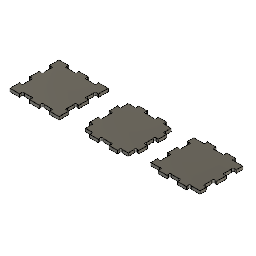
a5_box (Autodesk Fusion 360 design; units mm, degrees)
Autodesk Fusion 360 part; units mm, degrees
note: some values were not read from the file. Set by a fixed rule: which sketch regions a step uses.
sketch "Sketch1" plane through (0, 0, 0) normal (0, 0, 1) x (1, 0, 0)
  line L0 (-100.34, 0) -> (0, 0)
  line L1 (0, 0) -> (0, 70.41)
  line L2 (0, 70.41) -> (-100.34, 70.41)
  line L3 (-100.34, 70.41) -> (-100.34, 0)
  dimension "d1" = 100.34
  dimension "d2" = 70.41
  constraint horizontal L0
  constraint vertical L1
  constraint horizontal L2
  constraint vertical L3
  constraint coincident L0.end L1.start
  measures "d1" distance of L0.start L0.end
  measures "d2" distance of L0.start L2.end
  measures "d104" distance of L0.end
extrude "Extrude1" add sketch "Sketch1" along normal blind 1.58 makes body 1
sketch "Sketch3" plane through (0, 0, 0) normal (0, 0, 1) x (1, 0, 0)
  line L0 (10, 25) -> (35, 25)
  line L1 (35, 25) -> (35, 0)
  line L2 (35, 0) -> (10, 0)
  line L3 (10, 0) -> (10, 25)
  line L4 (10, 25) -> (11.58, 25)
  line L5 (11.58, 25) -> (11.58, 0)
  line L6 (11.58, 0) -> (10, 0)
  line L7 (10, 0) -> (10, 25)
  line L8 (10, 25) -> (35, 25)
  line L9 (35, 25) -> (35, 23.42)
  line L10 (35, 23.42) -> (10, 23.42)
  line L11 (10, 23.42) -> (10, 25)
  line L12 (35, 25) -> (33.42, 25)
  line L13 (33.42, 25) -> (33.42, 0)
  line L14 (33.42, 0) -> (35, 0)
  line L15 (35, 0) -> (35, 25)
  line L16 (10, 0) -> (35, 0)
  line L17 (35, 0) -> (35, 1.58)
  line L18 (35, 1.58) -> (10, 1.58)
  line L19 (10, 1.58) -> (10, 0)
  dimension "d5" = 25
  dimension "d6" = 25
  dimension "d14" = 1.58
  dimension "d15" = 1.58
  dimension "d16" = 1.58
  dimension "d17" = 1.58
  constraint horizontal L0
  constraint vertical L1
  constraint horizontal L2
  constraint vertical L3
  constraint horizontal L4
  constraint vertical L5
  constraint horizontal L6
  constraint vertical L7
  constraint horizontal L8
  constraint vertical L9
  constraint horizontal L10
  constraint vertical L11
  constraint horizontal L12
  constraint vertical L13
  constraint horizontal L14
  constraint vertical L15
  constraint horizontal L16
  constraint vertical L17
  constraint horizontal L18
  constraint vertical L19
  measures "d5" distance of L0.start L0.end
  measures "d6" distance of L0.start L2.end
  measures "d14" distance of L0.start L4.end
  measures "d15" distance of L0.start L10.end
  measures "d16" distance of L0.end L12.end
  measures "d17" distance of L2.end L18.end
extrude "Extrude3" add sketch "Sketch3" along normal blind 25 separate body contours L0 L3 L4 L5 L7 L8 L10 L11 | L0 L5 L8 L10 L13 | L3 L5 L7 L10 L18 | L0 L1 L8 L9 L10 L12 L13 L15 | L2 L3 L5 L6 L7 L16 L18 L19 | L1 L10 L13 L15 L18 | L2 L5 L13 L16 L18 | L1 L2 L13 L14 L15 L16 L17 L18 makes body 2
extrude "Extrude4" add sketch "Sketch3" along normal blind 1.58 contours L5 L10 L13 L18 bodies 2
sketch "Sketch5" plane through (0, 0, 25) normal (0, 0, 1) x (-1, 0, 0)
  line L0 (-11.58, -1.58) -> (-11.58, -23.42)
  line L1 (-11.58, -23.42) -> (-33.42, -23.42)
  line L2 (-33.42, -23.42) -> (-33.42, -1.58)
  line L3 (-33.42, -1.58) -> (-11.58, -1.58)
  line L4 (-10, -25) -> (-10, 0)
  line L5 (-10, 0) -> (-35, 0)
  line L6 (-35, 0) -> (-35, -25)
  line L7 (-35, -25) -> (-10, -25)
  line L8 (-10, -25) -> (-35, -25)
  line L9 (-35, -25) -> (-35, 0)
  line L10 (-35, 0) -> (-10, 0)
  line L11 (-10, 0) -> (-10, -25)
  constraint horizontal L8
  constraint vertical L9
  constraint horizontal L10
  constraint vertical L11
  constraint coincident L5.end L6.start
  constraint coincident L4.start L7.end
extrude "Extrude5" add sketch "Sketch5" against normal blind 1.58 contours L0 L1 L2 L3 bodies 2
sketch "Sketch6" plane through (0, 0, 25) normal (0, 0, 1) x (-1, 0, 0)
  line L0 (-10, -25) -> (-10, 0)
  line L1 (-10, 0) -> (-35, 0)
  line L2 (-35, 0) -> (-35, -25)
  line L3 (-35, -25) -> (-10, -25)
  line L4 (-14.9996, 0) -> (-14.9996, -1.58)
  line L5 (-19.9996, -1.58) -> (-19.9996, 0)
  line L6 (-25.0019, 0) -> (-25.0019, -1.58)
  line L7 (-30.0019, -1.58) -> (-30.0019, 0)
  line L8 (-14.9996, -1.58) -> (-19.9996, -1.58)
  line L9 (-25.0019, -1.58) -> (-30.0019, -1.58)
  line L10 (-11.58, -1.58) -> (-33.42, -1.58)
  line L11 (-14.7996, 0) -> (-14.7996, -1.78)
  line L12 (-14.7996, -1.78) -> (-20.1996, -1.78)
  line L13 (-20.1996, -1.78) -> (-20.1996, 0)
  line L14 (-24.8, 0) -> (-24.8, -1.78)
  line L15 (-24.8, -1.78) -> (-30.2, -1.78)
  line L16 (-30.2, -1.78) -> (-30.2, 0)
  line L17 (-55.1361, -25) -> (-80.1361, -25)
  line L18 (-80.1361, -25) -> (-80.1361, 0)
  line L19 (-80.1361, 0) -> (-55.1361, 0)
  line L20 (-55.1361, 0) -> (-55.1361, -25)
  line L21 (-60.1361, 0) -> (-65.1361, 0)
  line L22 (-65.1361, 0) -> (-65.1361, -1.58)
  line L23 (-65.1361, -1.58) -> (-60.1361, -1.58)
  line L24 (-60.1361, -1.58) -> (-60.1361, 0)
  line L25 (-70.1361, 0) -> (-75.1361, 0)
  line L26 (-75.1361, 0) -> (-75.1361, -1.58)
  line L27 (-75.1361, -1.58) -> (-70.1361, -1.58)
  line L28 (-70.1361, -1.58) -> (-70.1361, 0)
  line L29 (-67.6361, -25) -> (-67.6361, 0) construction
  line L30 (-55.1361, -12.5) -> (-80.1361, -12.5) construction
  line L31 (-70.1361, -23.42) -> (-70.1361, -25)
  line L32 (-75.1361, -23.42) -> (-70.1361, -23.42)
  line L33 (-75.1361, -25) -> (-75.1361, -23.42)
  line L34 (-65.1361, -25) -> (-65.1361, -23.42)
  line L35 (-65.1361, -23.42) -> (-60.1361, -23.42)
  line L36 (-60.1361, -23.42) -> (-60.1361, -25)
  line L37 (-55.1361, -25) -> (-80.1361, 0) construction
  line L38 (-80.1361, -25) -> (-55.1361, 0) construction
  line L39 (-55.1361, -5) -> (-56.7161, -5)
  line L40 (-55.1361, -15) -> (-56.7161, -15)
  line L41 (-56.7161, -20) -> (-55.1361, -20)
  line L42 (-56.7161, -15) -> (-56.7161, -20)
  line L43 (-56.7161, -10) -> (-55.1361, -10)
  line L44 (-56.7161, -5) -> (-56.7161, -10)
  line L45 (-80.1361, -10) -> (-78.5561, -10)
  line L46 (-78.5561, -5) -> (-80.1361, -5)
  line L47 (-78.5561, -10) -> (-78.5561, -5)
  line L48 (-80.1361, -20) -> (-78.5561, -20)
  line L49 (-78.5561, -20) -> (-78.5561, -15)
  line L50 (-78.5561, -15) -> (-80.1361, -15)
  point P0 (-55.1361, -12.5)
  point P1 (-80.1361, -12.5)
  dimension "d24" = 1.78
  dimension "d25" = 0.2
  dimension "d26" = 5
  dimension "d27" = 5.4
  dimension "d28" = 1.78
  dimension "d29" = 5
  dimension "d30" = 5.4
  dimension "d31" = 25
  dimension "d32" = 25
  dimension "d33" = 5
  dimension "d34" = 1.58
  dimension "d35" = 5
  dimension "d36" = 1.58
  dimension "d37" = 5
  dimension "d38" = 5
  constraint coincident L1 L4.start
  constraint coincident L1 L5.end
  constraint perpendicular L1 L5
  constraint coincident L1 L6.start
  constraint coincident L1 L7.end
  constraint perpendicular L1 L7
  constraint perpendicular L5 L8
  constraint perpendicular L7 L9
  constraint coincident L4.end L10
  constraint coincident L6.end L10
  constraint perpendicular L6 L9
  constraint perpendicular L4 L8
  constraint coincident L1 L11.start
  constraint perpendicular L10 L11
  constraint perpendicular L11 L12
  constraint coincident L1 L13.end
  constraint perpendicular L1 L13
  constraint coincident L1 L14.start
  constraint perpendicular L10 L14
  constraint perpendicular L14 L15
  constraint coincident L1 L16.end
  constraint perpendicular L1 L16
  constraint horizontal L17
  constraint vertical L18
  constraint horizontal L19
  constraint vertical L20
  constraint horizontal L21
  constraint vertical L22
  constraint horizontal L23
  constraint vertical L24
  constraint coincident L19 L21.start
  constraint horizontal L25
  constraint vertical L26
  constraint horizontal L27
  constraint vertical L28
  constraint coincident L19 L25.start
  constraint midpoint L17 L29.start
  constraint midpoint L19 L29.end
  constraint midpoint L20 P0
  constraint midpoint L18 P1
  constraint symmetric L21.start L30 L36.end
  constraint symmetric L21.end L30 L34.start
  constraint symmetric L22.end L30 L34.end
  constraint symmetric L23.end L30 L35.end
  constraint symmetric L25.start L30 L31.end
  constraint symmetric L25.end L30 L33.start
  constraint symmetric L26.end L30 L32.start
  constraint symmetric L27.end L30 L31.start
  constraint symmetric L29.start L37 P0
  constraint symmetric L31.start L37 L43.start
  constraint symmetric L31.end L37 L43.end
  constraint symmetric L32.start L37 L39.end
  constraint symmetric L33.start L37 L39.start
  constraint symmetric L34.start L37 L40.start
  constraint symmetric L34.end L37 L40.end
  constraint symmetric L35.end L37 L41.start
  constraint symmetric L36.end L37 L41.end
  constraint symmetric L29.start L38 P1
  constraint symmetric L31.start L38 L49.end
  constraint symmetric L31.end L38 L50.end
  constraint symmetric L32.start L38 L48.end
  constraint symmetric L33.start L38 L48.start
  constraint symmetric L34.start L38 L45.start
  constraint symmetric L34.end L38 L45.end
  constraint symmetric L35.end L38 L46.start
  constraint symmetric L36.end L38 L46.end
  measures "d24" distance of L11.start L11.end
  measures "d25" distance of L4 L11
  measures "d26" distance of L4.end L5.start
  measures "d27" distance of L11.end L12.end
  measures "d28" distance of L14.start L14.end
  measures "d29" distance of L6.end L7.start
  measures "d30" distance of L14.end L15.end
  measures "d31" distance of L17.start L17.end
  measures "d32" distance of L17.start L19.end
  measures "d33" distance of L21.start L21.end
  measures "d34" distance of L21.start L23.end
  measures "d35" distance of L20 L24
  measures "d36" distance of L25.start L27.end
  measures "d37" distance of L25.start L25.end
  measures "d38" distance of L22 L28
extrude "Extrude6" add sketch "Sketch6" along normal blind 1.58 separate body contours L17 L18 L19 L20 L22 L23 L24 L26 L27 L28 L31 L32 L33 L34 L35 L36 L39 L40 L41 L42 L43 L44 L45 L46 L47 L48 L49 L50 makes body 3
sketch "Sketch9" plane through (0, 0, 26.58) normal (0, 0, 1) x (-1, 0, 0)
  line L0 (-75.1361, -25) -> (-75.1361, -23.42)
  line L1 (-75.1361, -23.42) -> (-70.1361, -23.42)
  line L2 (-70.1361, -23.42) -> (-70.1361, -25)
  line L3 (-70.1361, -25) -> (-65.1361, -25)
  line L4 (-65.1361, -25) -> (-65.1361, -23.42)
  line L5 (-65.1361, -23.42) -> (-60.1361, -23.42)
  line L6 (-60.1361, -23.42) -> (-60.1361, -25)
  line L7 (-60.1361, -25) -> (-55.1361, -25)
  line L8 (-55.1361, -25) -> (-55.1361, -20)
  line L9 (-55.1361, -20) -> (-56.7161, -20)
  line L10 (-56.7161, -20) -> (-56.7161, -15)
  line L11 (-56.7161, -15) -> (-55.1361, -15)
  line L12 (-55.1361, -15) -> (-55.1361, -10)
  line L13 (-55.1361, -10) -> (-56.7161, -10)
  line L14 (-56.7161, -10) -> (-56.7161, -5)
  line L15 (-56.7161, -5) -> (-55.1361, -5)
  line L16 (-55.1361, -5) -> (-55.1361, 0)
  line L17 (-55.1361, 0) -> (-60.1361, 0)
  line L18 (-60.1361, 0) -> (-60.1361, -1.58)
  line L19 (-60.1361, -1.58) -> (-65.1361, -1.58)
  line L20 (-65.1361, -1.58) -> (-65.1361, 0)
  line L21 (-65.1361, 0) -> (-70.1361, 0)
  line L22 (-70.1361, 0) -> (-70.1361, -1.58)
  line L23 (-70.1361, -1.58) -> (-75.1361, -1.58)
  line L24 (-75.1361, -1.58) -> (-75.1361, 0)
  line L25 (-75.1361, 0) -> (-80.1361, 0)
  line L26 (-80.1361, 0) -> (-80.1361, -5)
  line L27 (-80.1361, -5) -> (-78.5561, -5)
  line L28 (-78.5561, -5) -> (-78.5561, -10)
  line L29 (-78.5561, -10) -> (-80.1361, -10)
  line L30 (-80.1361, -10) -> (-80.1361, -15)
  line L31 (-80.1361, -15) -> (-78.5561, -15)
  line L32 (-78.5561, -15) -> (-78.5561, -20)
  line L33 (-78.5561, -20) -> (-80.1361, -20)
  line L34 (-80.1361, -20) -> (-80.1361, -25)
  line L35 (-80.1361, -25) -> (-75.1361, -25)
  line L36 (-60.1361, -23.42) -> (-61.3154, -24.5992) construction
  line L37 (-60.1361, -23.42) -> (-58.4685, -23.42) construction
  circle A0 centre (-60.5571, -23.8409) radius 0.5953
  line L38 (-62.6361, -23.42) -> (-62.6361, -1.58) construction
  line L39 (-67.6361, -25) -> (-67.6361, 0) construction
  line L40 (-55.1361, -12.5) -> (-80.1361, -12.5) construction
  line L41 (-80.1361, 0) -> (-55.1361, -25) construction
  circle A1 centre (-64.7152, -23.8409) radius 0.5953
  circle A2 centre (-74.7152, -23.8409) radius 0.5953
  circle A3 centre (-70.5571, -23.8409) radius 0.5953
  circle A4 centre (-60.5571, -1.1591) radius 0.5953
  circle A5 centre (-64.7152, -1.1591) radius 0.5953
  circle A6 centre (-70.5571, -1.1591) radius 0.5953
  circle A7 centre (-74.7152, -1.1591) radius 0.5953
  circle A8 centre (-56.2952, -19.5791) radius 0.5953
  circle A9 centre (-56.2952, -15.4209) radius 0.5953
  circle A10 centre (-56.2952, -9.5791) radius 0.5953
  circle A11 centre (-56.2952, -5.4209) radius 0.5953
  circle A12 centre (-78.9771, -15.4209) radius 0.5953
  circle A13 centre (-78.9771, -19.5791) radius 0.5953
  circle A14 centre (-78.9771, -9.5791) radius 0.5953
  circle A15 centre (-78.9771, -5.4209) radius 0.5953
  dimension "d41" = 135
  dimension "d42" = 1.1906
  dimension "d43" = 0.5953
  constraint horizontal L37
  constraint coincident L5.end L6.start
  constraint coincident L36 A0.centre
  constraint midpoint L5 L38.start
  constraint midpoint L19 L38.end
  constraint midpoint L3 L39.start
  constraint midpoint L21 L39.end
  constraint midpoint L12 L40.start
  constraint midpoint L30 L40.end
  constraint coincident L25.end L26.start
  constraint coincident L7.end L8.start
  constraint symmetric A0 L38 A1
  constraint symmetric A0 L39 A2
  constraint symmetric L39 A1 A3
  constraint symmetric A0 L40 A4
  constraint symmetric L40 A1 A5
  constraint symmetric L40 A2 A7
  constraint symmetric L40 A3 A6
  constraint symmetric A0 L41 A8
  constraint symmetric L41 A1 A9
  constraint symmetric L41 A2 A11
  constraint symmetric L41 A3 A10
  constraint symmetric L39 A8 A13
  constraint symmetric L39 A9 A12
  constraint symmetric L39 A10 A14
  constraint symmetric L39 A11 A15
  measures "d41" angle of L36 L37
  measures "d42" diameter of A0
  measures "d43" distance of L5.end A0.centre
extrude "Extrude7" cut sketch "Sketch9" against normal up to surface (1.58 mm away) contours L0 A2 | L0 L1 A2 | L1 A2 | L32 L33 A13 | L33 A13 | L1 A3 | L1 L2 A3 | L32 A13 | L2 A3 | L31 L32 A12 | L32 A12 | L31 A12 | L4 A1 | L4 L5 A1 | L5 A1 | L28 L29 A14 | L29 A14 | L28 A14 | L5 A0 | L5 L6 A0 | L27 L28 A15 | L28 A15 | L6 A0 | L27 A15 | L9 A8 | L9 L10 A8 | L23 L24 A7 | L24 A7 | L10 A8 | L23 A7 | L10 A9 | L10 L11 A9 | L22 L23 A6 | L23 A6 | L11 A9 | L22 A6 | L19 L20 A5 | L20 A5 | L13 A10 | L13 L14 A10 | L19 A5 | L14 A10 | L18 L19 A4 | L19 A4 | L14 A11 | L14 L15 A11 | L18 A4 | L15 A11 bodies 3
sketch "Sketch10" plane through (0, 0, 0) normal (0, 0, 1) x (1, 0, 0)
  line L0 (115.2, 23.42) -> (115.2, 0)
  line L1 (115.2, 0) -> (90.2, 0)
  line L2 (90.2, 0) -> (90.2, 19.6)
  line L3 (90.2, 25) -> (95.6, 25)
  line L4 (95.6, 25) -> (95.6, 23.42)
  line L5 (95.6, 23.42) -> (90.2, 23.42)
  line L6 (90.2, 23.42) -> (90.2, 25)
  line L7 (100, 25) -> (105.4, 25)
  line L8 (105.4, 25) -> (105.4, 23.42)
  line L9 (105.4, 23.42) -> (100, 23.42)
  line L10 (100, 23.42) -> (100, 25)
  line L11 (109.8, 25) -> (115.2, 25)
  line L12 (115.2, 25) -> (115.2, 23.42)
  line L13 (115.2, 23.42) -> (109.8, 23.42)
  line L14 (109.8, 23.42) -> (109.8, 25)
  line L15 (90.2, 12.5) -> (115.2, 12.5) construction
  line L16 (102.7, 25) -> (102.7, 0) construction
  line L17 (91.78, 5.4) -> (91.78, 0)
  line L18 (90.2, 5.4) -> (91.78, 5.4)
  line L19 (91.78, 9.8) -> (90.2, 9.8)
  line L20 (91.78, 15.2) -> (91.78, 9.8)
  line L21 (90.2, 15.2) -> (91.78, 15.2)
  line L22 (91.78, 19.6) -> (90.2, 19.6)
  line L23 (91.78, 25) -> (91.78, 19.6)
  line L24 (109.8, 1.58) -> (115.2, 1.58)
  line L25 (109.8, 0) -> (109.8, 1.58)
  line L26 (105.4, 1.58) -> (105.4, 0)
  line L27 (100, 1.58) -> (105.4, 1.58)
  line L28 (100, 0) -> (100, 1.58)
  line L29 (95.6, 1.58) -> (95.6, 0)
  line L30 (90.2, 1.58) -> (95.6, 1.58)
  line L31 (113.62, 19.6) -> (113.62, 25)
  line L32 (115.2, 19.6) -> (113.62, 19.6)
  line L33 (113.62, 15.2) -> (115.2, 15.2)
  line L34 (113.62, 9.8) -> (113.62, 15.2)
  line L35 (115.2, 9.8) -> (113.62, 9.8)
  line L36 (113.62, 5.4) -> (115.2, 5.4)
  line L37 (113.62, 0) -> (113.62, 5.4)
  line L38 (90.2, 23.42) -> (90.2, 25)
  line L39 (90.2, 19.6) -> (90.2, 23.42)
  line L40 (115.2, 25) -> (115.2, 23.42)
  line L41 (109.8, 25) -> (115.2, 25)
  line L42 (105.4, 25) -> (109.8, 25)
  line L43 (90.2, 25) -> (95.6, 25)
  line L44 (100, 25) -> (105.4, 25)
  line L45 (95.6, 25) -> (100, 25)
  point P0 (102.7, 12.5)
  dimension "d46" = 25
  dimension "d47" = 25
  dimension "d48" = 5.4
  dimension "d49" = 1.58
  dimension "d50" = 5.4
  dimension "d51" = 1.58
  dimension "d52" = 5.4
  dimension "d53" = 1.58
  dimension "d57" = 360
  dimension "d73" = 4.4
  dimension "d74" = 4.4
  constraint horizontal L43
  constraint vertical L0
  constraint horizontal L1
  constraint vertical L2
  constraint horizontal L3
  constraint vertical L4
  constraint horizontal L5
  constraint vertical L6
  constraint horizontal L7
  constraint vertical L8
  constraint horizontal L9
  constraint vertical L10
  constraint coincident L7.start L43
  constraint horizontal L11
  constraint vertical L12
  constraint horizontal L13
  constraint vertical L14
  constraint coincident L11.start L43
  constraint midpoint L1 L16.end
  constraint midpoint L16 P0
  constraint collinear L0 L12
  constraint coincident L2 L15.start
  constraint coincident L0 L15.end
  constraint coincident L16.start L43
  measures "d46" distance of L3.start L11.end
  measures "d47" distance of L3.start L1.end
  measures "d48" distance of L3.start L3.end
  measures "d49" distance of L3.start L5.end
  measures "d50" distance of L7.start L7.end
  measures "d51" distance of L7.start L9.end
  measures "d52" distance of L11.start L11.end
  measures "d53" distance of L11.start L13.end
  measures "d73" distance of L4 L10
  measures "d74" distance of L8 L14
extrude "Extrude8" add sketch "Sketch10" along normal blind 1.58 separate body contours L0 L1 L2 L4 L5 L8 L9 L10 L13 L14 L17 L18 L19 L20 L21 L22 L23 L24 L25 L26 L27 L28 L29 L30 L31 L32 L33 L34 L35 L36 L37 L42 L45 makes body 4
sketch "Sketch12" plane through (0, 0, 0) normal (0, 0, 1) x (1, 0, 0)
  line L0 (100, 23.42) -> (100, 25) construction
  circle A0 centre (114.041, 20.0209) radius 0.5953
  circle A1 centre (91.3591, 20.0209) radius 0.5953
  line L1 (95.6, 23.42) -> (97.2763, 23.42) construction
  line L2 (102.7, 25.8483) -> (102.7, 0.1169) construction
  circle A2 centre (104.9791, 23.8409) radius 0.5953
  circle A3 centre (114.041, 4.9791) radius 0.5953
  circle A4 centre (110.221, 1.1591) radius 0.5953
  circle A5 centre (100.421, 1.1591) radius 0.5953
  circle A6 centre (91.3591, 4.9791) radius 0.5953
  circle A7 centre (91.3591, 10.2209) radius 0.5953
  circle A8 centre (114.041, 10.2209) radius 0.5953
  circle A9 centre (114.041, 14.7791) radius 0.5953
  line L3 (95.6, 23.42) -> (93.7059, 25.3141) construction
  circle A10 centre (95.1791, 23.8409) radius 0.5953
  circle A11 centre (91.3591, 14.7791) radius 0.5953
  circle A12 centre (104.9791, 1.1591) radius 0.5953
  line L4 (95.6, 25) -> (100, 25) construction
  circle A13 centre (100.421, 23.8409) radius 0.5953
  line L5 (97.8, 25) -> (97.8, -1.1306) construction
  circle A14 centre (110.221, 23.8409) radius 0.5953
  circle A15 centre (95.1791, 1.1591) radius 0.5953
  line L6 (102.7, 25) -> (102.7, 0)
  point P0 (102.7, 12.5)
  point P1 (95.6, 25)
  point P2 (100, 25)
  point P3 (102.7, 12.5)
  point P4 (95.6, 23.42)
  point P5 (102.7, 12.5)
  point P6 (95.6, 25)
  point P7 (95.6, 23.42)
  dimension "d66" = 360
  dimension "d67" = 135
  dimension "d68" = 1.1906
  dimension "d72" = 0.5953
  constraint horizontal L1
  constraint coincident A10.centre L3
  constraint coincident P6 P1
  constraint coincident P2 L0.end
  constraint midpoint L5.start L4
  constraint perpendicular L4 L5
  constraint symmetric A10 A13 L5
  constraint symmetric L2 A10 A14
  constraint symmetric L2 A2 A13
  constraint coincident P5 P3
  constraint collinear L2 L6
  constraint coincident P7 P4
  measures "d67" angle of L1 L3
  measures "d68" diameter of A10
  measures "d72" distance of A10.centre P7
extrude "Extrude9" cut sketch "Sketch12" along normal up to surface (1.58 mm away) bodies 4
move_body "Move1" bodies 3 to x (1, 0, 0) y (0, 1, 0) z (0, 0, 1) at (0, 0, -25)
sketch "Sketch17" plane through (0, 0, 1.58) normal (0, 0, 1) x (-1, 0, 0)
  arc A0 (-90.9381, -9.8) -> (-91.78, -10.6419) centre (-91.3591, -10.2209) ccw
  line L0 (-90.9381, -9.8) -> (-90.2, -9.8)
  line L1 (-90.2, -9.8) -> (-90.2, -5.4)
  line L2 (-90.2, -5.4) -> (-90.9381, -5.4)
  arc A1 (-91.78, -4.5581) -> (-90.9381, -5.4) centre (-91.3591, -4.9791) ccw
  line L3 (-91.78, -4.5581) -> (-91.78, -1.58)
  line L4 (-91.78, -1.58) -> (-94.7581, -1.58)
  arc A2 (-95.6, -0.7381) -> (-94.7581, -1.58) centre (-95.1791, -1.1591) ccw
  line L5 (-95.6, -0.7381) -> (-95.6, 0)
  line L6 (-95.6, 0) -> (-100, 0)
  line L7 (-100, 0) -> (-100, -0.7381)
  arc A3 (-100.8419, -1.58) -> (-100, -0.7381) centre (-100.421, -1.1591) ccw
  line L8 (-100.8419, -1.58) -> (-104.5581, -1.58)
  arc A4 (-105.4, -0.7381) -> (-104.5581, -1.58) centre (-104.9791, -1.1591) ccw
  line L9 (-105.4, -0.7381) -> (-105.4, 0)
  line L10 (-105.4, 0) -> (-109.8, 0)
  line L11 (-109.8, 0) -> (-109.8, -0.7381)
  arc A5 (-110.6419, -1.58) -> (-109.8, -0.7381) centre (-110.221, -1.1591) ccw
  line L12 (-110.6419, -1.58) -> (-113.62, -1.58)
  line L13 (-113.62, -1.58) -> (-113.62, -4.5581)
  arc A6 (-114.4619, -5.4) -> (-113.62, -4.5581) centre (-114.041, -4.9791) ccw
  line L14 (-114.4619, -5.4) -> (-115.2, -5.4)
  line L15 (-115.2, -5.4) -> (-115.2, -9.8)
  line L16 (-115.2, -9.8) -> (-114.4619, -9.8)
  arc A7 (-113.62, -10.6419) -> (-114.4619, -9.8) centre (-114.041, -10.2209) ccw
  line L17 (-113.62, -10.6419) -> (-113.62, -14.3581)
  arc A8 (-114.4619, -15.2) -> (-113.62, -14.3581) centre (-114.041, -14.7791) ccw
  line L18 (-114.4619, -15.2) -> (-115.2, -15.2)
  line L19 (-115.2, -15.2) -> (-115.2, -19.6)
  line L20 (-115.2, -19.6) -> (-114.4619, -19.6)
  arc A9 (-113.62, -20.4419) -> (-114.4619, -19.6) centre (-114.041, -20.0209) ccw
  line L21 (-113.62, -20.4419) -> (-113.62, -23.42)
  line L22 (-113.62, -23.42) -> (-110.6419, -23.42)
  arc A10 (-109.8, -24.2619) -> (-110.6419, -23.42) centre (-110.221, -23.8409) ccw
  line L23 (-109.8, -24.2619) -> (-109.8, -25)
  line L24 (-105.4, -25) -> (-105.4, -24.2619)
  arc A11 (-104.5581, -23.42) -> (-105.4, -24.2619) centre (-104.9791, -23.8409) ccw
  line L25 (-104.5581, -23.42) -> (-100.8419, -23.42)
  arc A12 (-100, -24.2619) -> (-100.8419, -23.42) centre (-100.421, -23.8409) ccw
  line L26 (-100, -24.2619) -> (-100, -25)
  line L27 (-95.6, -25) -> (-95.6, -24.2619)
  arc A13 (-94.7581, -23.42) -> (-95.6, -24.2619) centre (-95.1791, -23.8409) ccw
  line L28 (-94.7581, -23.42) -> (-91.78, -23.42)
  line L29 (-91.78, -23.42) -> (-91.78, -20.4419)
  arc A14 (-90.9381, -19.6) -> (-91.78, -20.4419) centre (-91.3591, -20.0209) ccw
  line L30 (-90.9381, -19.6) -> (-90.2, -19.6)
  line L31 (-90.2, -19.6) -> (-90.2, -15.2)
  line L32 (-90.2, -15.2) -> (-90.9381, -15.2)
  arc A15 (-91.78, -14.3581) -> (-90.9381, -15.2) centre (-91.3591, -14.7791) ccw
  line L33 (-91.78, -14.3581) -> (-91.78, -10.6419)
  line L34 (-125, 0) -> (-150, 0)
  line L35 (-150, 0) -> (-150, -25)
  line L36 (-150, -25) -> (-125, -25)
  line L37 (-125, -25) -> (-125, 0)
  line L38 (-109.8, -25) -> (-105.4, -25)
  line L39 (-100, -25) -> (-95.6, -25)
  line L40 (-125, -25) -> (-130.3, -25)
  line L41 (-130.3, -25) -> (-130.3, -23.42)
  line L42 (-130.3, -23.42) -> (-125, -23.42)
  line L43 (-125, -23.42) -> (-125, -25)
  line L44 (-134.85, -25) -> (-140.15, -25)
  line L45 (-140.15, -25) -> (-140.15, -23.42)
  line L46 (-140.15, -23.42) -> (-134.85, -23.42)
  line L47 (-134.85, -23.42) -> (-134.85, -25)
  line L48 (-150, -25) -> (-144.7, -25)
  line L49 (-144.7, -25) -> (-144.7, -23.42)
  line L50 (-144.7, -23.42) -> (-150, -23.42)
  line L51 (-150, -23.42) -> (-150, -25)
  line L52 (-125, -12.5) -> (-150, -12.5) construction
  line L53 (-130.3, -1.58) -> (-125, -1.58)
  line L54 (-130.3, 0) -> (-130.3, -1.58)
  line L55 (-134.85, -1.58) -> (-134.85, 0)
  line L56 (-140.15, -1.58) -> (-134.85, -1.58)
  line L57 (-140.15, 0) -> (-140.15, -1.58)
  line L58 (-144.7, 0) -> (-144.7, -1.58)
  line L59 (-144.7, -1.58) -> (-150, -1.58)
  line L60 (-125, -20) -> (-126.58, -20)
  line L61 (-126.58, -20) -> (-126.58, -15)
  line L62 (-126.58, -15) -> (-125, -15)
  line L63 (-125, -15) -> (-125, -20)
  line L64 (-125, -10) -> (-126.58, -10)
  line L65 (-126.58, -10) -> (-126.58, -5)
  line L66 (-126.58, -5) -> (-125, -5)
  line L67 (-125, -5) -> (-125, -10)
  line L68 (-137.5, -25) -> (-137.5, 0) construction
  line L69 (-150, -20) -> (-148.42, -20)
  line L70 (-148.42, -20) -> (-148.42, -15)
  line L71 (-148.42, -15) -> (-150, -15)
  line L72 (-150, -10) -> (-148.42, -10)
  line L73 (-148.42, -10) -> (-148.42, -5)
  line L74 (-148.42, -5) -> (-150, -5)
  dimension "d75" = 25
  dimension "d76" = 25
  dimension "d98" = 1.58
  dimension "d99" = 5.3
  dimension "d100" = 5.3
  dimension "d101" = 1.58
  dimension "d102" = 5.3
  dimension "d103" = 1.58
  dimension "d104" = 4.55
  dimension "d105" = 5
  dimension "d106" = 1.58
  dimension "d107" = 5
  dimension "d108" = 5
  dimension "d109" = 1.58
  dimension "d110" = 5
  constraint horizontal L34
  constraint vertical L35
  constraint horizontal L36
  constraint vertical L37
  constraint horizontal L40
  constraint vertical L41
  constraint horizontal L42
  constraint vertical L43
  constraint horizontal L44
  constraint vertical L45
  constraint horizontal L46
  constraint vertical L47
  constraint coincident L36 L44.start
  constraint horizontal L48
  constraint vertical L49
  constraint horizontal L50
  constraint vertical L51
  constraint midpoint L37 L52.start
  constraint midpoint L35 L52.end
  constraint symmetric L40.end L52 L54.start
  constraint symmetric L41.end L52 L53.start
  constraint symmetric L42.end L52 L53.end
  constraint symmetric L44.start L52 L55.end
  constraint symmetric L44.end L52 L57.start
  constraint symmetric L45.end L52 L56.start
  constraint symmetric L46.end L52 L55.start
  constraint symmetric L48.end L52 L58.start
  constraint symmetric L49.end L52 L58.end
  constraint symmetric L50.end L52 L59.end
  constraint horizontal L60
  constraint vertical L61
  constraint horizontal L62
  constraint vertical L63
  constraint coincident L37 L60.start
  constraint horizontal L64
  constraint vertical L65
  constraint horizontal L66
  constraint vertical L67
  constraint coincident L37 L64.start
  constraint midpoint L36 L68.start
  constraint midpoint L34 L68.end
  constraint symmetric L60.start L68 L69.start
  constraint symmetric L60.end L68 L69.end
  constraint symmetric L61.end L68 L70.end
  constraint symmetric L62.end L68 L71.end
  constraint symmetric L64.start L68 L72.start
  constraint symmetric L64.end L68 L72.end
  constraint symmetric L65.end L68 L73.end
  constraint symmetric L66.end L68 L74.end
  measures "d75" distance of L34.start L34.end
  measures "d76" distance of L34.start L36.end
  measures "d98" distance of L36.end L42.end
  measures "d99" distance of L36.end L40.end
  measures "d100" distance of L44.start L44.end
  measures "d101" distance of L44.start L46.end
  measures "d102" distance of L35.end L48.end
  measures "d103" distance of L35.end L50.end
  measures "d104" distance of L41.end L46.end
  measures "d105" distance of L60.start L62.end
  measures "d106" distance of L60.start L60.end
  measures "d107" distance of L36 L60
  measures "d108" distance of L64.start L66.end
  measures "d109" distance of L64.start L64.end
  measures "d110" distance of L34 L66
sketch "Sketch18" plane through (0, 0, 1.58) normal (0, 0, 1) x (-1, 0, 0)
  line L0 (-144.7, -1.58) -> (-146.4461, 0.1661) construction
  line L1 (-144.7, -1.58) -> (-142.2306, -1.58) construction
  circle A0 centre (-145.121, -1.1591) radius 0.5953
  line L2 (-140.15, -25) -> (-140.15, -23.42) construction
  line L3 (-144.7, -25) -> (-140.15, -25) construction
  line L4 (-125, 0) -> (-150, 0) construction
  line L5 (-142.425, -25) -> (-142.425, 0) construction
  circle A1 centre (-139.7291, -1.1591) radius 0.5953
  line L6 (-137.5, -25) -> (-137.5, 0) construction
  circle A2 centre (-135.271, -1.1591) radius 0.5953
  circle A3 centre (-129.8791, -1.1591) radius 0.5953
  line L7 (-125, -12.5) -> (-150, -12.5) construction
  circle A4 centre (-129.8791, -23.8409) radius 0.5953
  circle A5 centre (-135.271, -23.8409) radius 0.5953
  circle A6 centre (-139.7291, -23.8409) radius 0.5953
  circle A7 centre (-145.121, -23.8409) radius 0.5953
  line L8 (-126.58, -20) -> (-125.0395, -18.4595) construction
  line L9 (-126.58, -20) -> (-124.4014, -20) construction
  circle A8 centre (-126.1591, -19.5791) radius 0.5953
  line L10 (-125, -15) -> (-125, -20) construction
  line L11 (-150, 0) -> (-150, -25) construction
  line L12 (-125, -17.5) -> (-150, -17.5) construction
  circle A9 centre (-126.1591, -15.4209) radius 0.5953
  circle A10 centre (-126.1591, -9.5791) radius 0.5953
  circle A11 centre (-126.1591, -5.4209) radius 0.5953
  circle A12 centre (-148.841, -19.5791) radius 0.5953
  circle A13 centre (-148.841, -15.4209) radius 0.5953
  circle A14 centre (-148.841, -9.5791) radius 0.5953
  circle A15 centre (-148.841, -5.4209) radius 0.5953
  point P0 (-144.7, -1.58)
  point P1 (-144.7, -25)
  point P2 (-140.15, -25)
  point P3 (-125, -25)
  point P4 (-126.58, -20)
  dimension "d111" = 135
  dimension "d112" = 1.1906
  dimension "d113" = 0.5953
  dimension "d114" = 45
  dimension "d115" = 1.1906
  dimension "d116" = 0.5953
  constraint horizontal L1
  constraint coincident P0 L0.start
  constraint coincident L0 A0.centre
  constraint coincident P1 L3.start
  constraint coincident P2 L2.start
  constraint midpoint L3 L5.start
  constraint coincident L4 L5.end
  constraint perpendicular L3 L5
  constraint symmetric A0 L5 A1
  constraint symmetric A0 L6 A3
  constraint symmetric A1 L6 A2
  constraint symmetric A0 L7 A7
  constraint symmetric A1 L7 A6
  constraint symmetric A2 L7 A5
  constraint symmetric A3 L7 A4
  constraint horizontal L9
  constraint coincident P4 L8.start
  constraint coincident L8 A8.centre
  constraint midpoint L10 L12.start
  constraint coincident L11 L12.end
  constraint perpendicular L11 L12
  constraint symmetric A8 L12 A9
  constraint symmetric L7 A8 A11
  constraint symmetric L7 A9 A10
  constraint symmetric L6 A8 A12
  constraint symmetric L6 A9 A13
  constraint symmetric L6 A10 A14
  constraint symmetric L6 A11 A15
  measures "d111" angle of L0 L1
  measures "d112" diameter of A0
  measures "d113" distance of P0 A0.centre
  measures "d114" angle of L8 L9
  measures "d115" diameter of A8
  measures "d116" distance of P4 A8.centre
extrude "Extrude10" add sketch "Sketch17" along normal blind 1.58 separate body contours L34 L35 L36 L37 L41 L42 L45 L46 L47 L49 L50 L53 L54 L55 L56 L57 L58 L59 L60 L61 L62 L64 L65 L66 L69 L70 L71 L72 L73 L74 makes body 5
extrude "Extrude11" cut sketch "Sketch18" along normal up to surface (1.58 mm away) bodies 5
sketch "Sketch19" plane through (0, 0, 1.58) normal (0, 0, 1) x (-1, 0, 0)
  arc A0 (-90.9381, -9.8) -> (-91.78, -10.6419) centre (-91.3591, -10.2209) ccw
  line L0 (-90.9381, -9.8) -> (-90.2, -9.8)
  line L1 (-90.2, -9.8) -> (-90.2, -5.4)
  line L2 (-90.2, -5.4) -> (-90.9381, -5.4)
  arc A1 (-91.78, -4.5581) -> (-90.9381, -5.4) centre (-91.3591, -4.9791) ccw
  line L3 (-91.78, -4.5581) -> (-91.78, -1.58)
  line L4 (-91.78, -1.58) -> (-94.7581, -1.58)
  arc A2 (-95.6, -0.7381) -> (-94.7581, -1.58) centre (-95.1791, -1.1591) ccw
  line L5 (-95.6, -0.7381) -> (-95.6, 0)
  line L6 (-95.6, 0) -> (-100, 0)
  line L7 (-100, 0) -> (-100, -0.7381)
  arc A3 (-100.8419, -1.58) -> (-100, -0.7381) centre (-100.421, -1.1591) ccw
  line L8 (-100.8419, -1.58) -> (-104.5581, -1.58)
  arc A4 (-105.4, -0.7381) -> (-104.5581, -1.58) centre (-104.9791, -1.1591) ccw
  line L9 (-105.4, -0.7381) -> (-105.4, 0)
  line L10 (-105.4, 0) -> (-109.8, 0)
  line L11 (-109.8, 0) -> (-109.8, -0.7381)
  arc A5 (-110.6419, -1.58) -> (-109.8, -0.7381) centre (-110.221, -1.1591) ccw
  line L12 (-110.6419, -1.58) -> (-113.62, -1.58)
  line L13 (-113.62, -1.58) -> (-113.62, -4.5581)
  arc A6 (-114.4619, -5.4) -> (-113.62, -4.5581) centre (-114.041, -4.9791) ccw
  line L14 (-114.4619, -5.4) -> (-115.2, -5.4)
  line L15 (-115.2, -5.4) -> (-115.2, -9.8)
  line L16 (-115.2, -9.8) -> (-114.4619, -9.8)
  arc A7 (-113.62, -10.6419) -> (-114.4619, -9.8) centre (-114.041, -10.2209) ccw
  line L17 (-113.62, -10.6419) -> (-113.62, -14.3581)
  arc A8 (-114.4619, -15.2) -> (-113.62, -14.3581) centre (-114.041, -14.7791) ccw
  line L18 (-114.4619, -15.2) -> (-115.2, -15.2)
  line L19 (-115.2, -15.2) -> (-115.2, -19.6)
  line L20 (-115.2, -19.6) -> (-114.4619, -19.6)
  arc A9 (-113.62, -20.4419) -> (-114.4619, -19.6) centre (-114.041, -20.0209) ccw
  line L21 (-113.62, -20.4419) -> (-113.62, -23.42)
  line L22 (-113.62, -23.42) -> (-110.6419, -23.42)
  arc A10 (-109.8, -24.2619) -> (-110.6419, -23.42) centre (-110.221, -23.8409) ccw
  line L23 (-109.8, -24.2619) -> (-109.8, -25)
  line L24 (-109.8, -25) -> (-105.4, -25)
  line L25 (-105.4, -25) -> (-105.4, -24.2619)
  arc A11 (-104.5581, -23.42) -> (-105.4, -24.2619) centre (-104.9791, -23.8409) ccw
  line L26 (-104.5581, -23.42) -> (-100.8419, -23.42)
  arc A12 (-100, -24.2619) -> (-100.8419, -23.42) centre (-100.421, -23.8409) ccw
  line L27 (-100, -24.2619) -> (-100, -25)
  line L28 (-100, -25) -> (-95.6, -25)
  line L29 (-95.6, -25) -> (-95.6, -24.2619)
  arc A13 (-94.7581, -23.42) -> (-95.6, -24.2619) centre (-95.1791, -23.8409) ccw
  line L30 (-94.7581, -23.42) -> (-91.78, -23.42)
  line L31 (-91.78, -23.42) -> (-91.78, -20.4419)
  arc A14 (-90.9381, -19.6) -> (-91.78, -20.4419) centre (-91.3591, -20.0209) ccw
  line L32 (-90.9381, -19.6) -> (-90.2, -19.6)
  line L33 (-90.2, -19.6) -> (-90.2, -15.2)
  line L34 (-90.2, -15.2) -> (-90.9381, -15.2)
  arc A15 (-91.78, -14.3581) -> (-90.9381, -15.2) centre (-91.3591, -14.7791) ccw
  line L35 (-91.78, -14.3581) -> (-91.78, -10.6419)
sketch "Sketch20" plane through (0, 0, 3.16) normal (0, 0, 1) x (-1, 0, 0)
  arc A0 (-126.58, -9.1581) -> (-125.7381, -10) centre (-126.1591, -9.5791) ccw
  line L0 (-126.58, -9.1581) -> (-126.58, -5.8419)
  arc A1 (-125.7381, -5) -> (-126.58, -5.8419) centre (-126.1591, -5.4209) ccw
  line L1 (-125.7381, -5) -> (-125, -5)
  line L2 (-125, -5) -> (-125, -1.58)
  line L3 (-125, -1.58) -> (-129.4581, -1.58)
  arc A2 (-130.3, -0.7381) -> (-129.4581, -1.58) centre (-129.8791, -1.1591) ccw
  line L4 (-130.3, -0.7381) -> (-130.3, 0)
  line L5 (-130.3, 0) -> (-134.85, 0)
  line L6 (-134.85, 0) -> (-134.85, -0.7381)
  arc A3 (-135.6919, -1.58) -> (-134.85, -0.7381) centre (-135.271, -1.1591) ccw
  line L7 (-135.6919, -1.58) -> (-139.3081, -1.58)
  arc A4 (-140.15, -0.7381) -> (-139.3081, -1.58) centre (-139.7291, -1.1591) ccw
  line L8 (-140.15, -0.7381) -> (-140.15, 0)
  line L9 (-140.15, 0) -> (-144.7, 0)
  line L10 (-144.7, 0) -> (-144.7, -0.7381)
  arc A5 (-145.5419, -1.58) -> (-144.7, -0.7381) centre (-145.121, -1.1591) ccw
  line L11 (-145.5419, -1.58) -> (-150, -1.58)
  line L12 (-150, -1.58) -> (-150, -5)
  line L13 (-150, -5) -> (-149.2619, -5)
  arc A6 (-148.42, -5.8419) -> (-149.2619, -5) centre (-148.841, -5.4209) ccw
  line L14 (-148.42, -5.8419) -> (-148.42, -9.1581)
  arc A7 (-149.2619, -10) -> (-148.42, -9.1581) centre (-148.841, -9.5791) ccw
  line L15 (-149.2619, -10) -> (-150, -10)
  line L16 (-150, -10) -> (-150, -15)
  line L17 (-150, -15) -> (-149.2619, -15)
  arc A8 (-148.42, -15.8419) -> (-149.2619, -15) centre (-148.841, -15.4209) ccw
  line L18 (-148.42, -15.8419) -> (-148.42, -19.1581)
  arc A9 (-149.2619, -20) -> (-148.42, -19.1581) centre (-148.841, -19.5791) ccw
  line L19 (-149.2619, -20) -> (-150, -20)
  line L20 (-150, -20) -> (-150, -23.42)
  line L21 (-150, -23.42) -> (-145.5419, -23.42)
  arc A10 (-144.7, -24.2619) -> (-145.5419, -23.42) centre (-145.121, -23.8409) ccw
  line L22 (-144.7, -24.2619) -> (-144.7, -25)
  line L23 (-144.7, -25) -> (-140.15, -25)
  line L24 (-140.15, -25) -> (-140.15, -24.2619)
  arc A11 (-139.3081, -23.42) -> (-140.15, -24.2619) centre (-139.7291, -23.8409) ccw
  line L25 (-139.3081, -23.42) -> (-135.6919, -23.42)
  arc A12 (-134.85, -24.2619) -> (-135.6919, -23.42) centre (-135.271, -23.8409) ccw
  line L26 (-134.85, -24.2619) -> (-134.85, -25)
  line L27 (-134.85, -25) -> (-130.3, -25)
  line L28 (-130.3, -25) -> (-130.3, -24.2619)
  arc A13 (-129.4581, -23.42) -> (-130.3, -24.2619) centre (-129.8791, -23.8409) ccw
  line L29 (-129.4581, -23.42) -> (-125, -23.42)
  line L30 (-125, -23.42) -> (-125, -20)
  line L31 (-125, -20) -> (-125.7381, -20)
  arc A14 (-126.58, -19.1581) -> (-125.7381, -20) centre (-126.1591, -19.5791) ccw
  line L32 (-126.58, -19.1581) -> (-126.58, -15.8419)
  arc A15 (-125.7381, -15) -> (-126.58, -15.8419) centre (-126.1591, -15.4209) ccw
  line L33 (-125.7381, -15) -> (-125, -15)
  line L34 (-125, -15) -> (-125, -10)
  line L35 (-125, -10) -> (-125.7381, -10)
hidden bodies 1 2
equation "d24 = 1.58 mm + 0.2 mm"
equation "d28 = 1.58 mm + 0.2 mm"
equation "d41 = 180 deg - 45 deg"
equation "d42 = ( 3 / 64 ) * 1 in"
equation "d43 = ( 3 / 128 ) * 1 in"
equation "d67 = 180 deg - 45 deg"
equation "d68 = ( 3 / 64 ) * 1 in"
equation "d72 = ( 3 / 128 ) * 1 in"
equation "d104 = ( ( 25 - 5.3 * 3 ) / 2 ) * 1 mm"
equation "d112 = ( 3 / 64 ) * 1 in"
equation "d113 = ( 3 / 128 ) * 1 in"
equation "d115 = ( 3 / 64 ) * 1 in"
equation "d116 = ( 3 / 128 ) * 1 in"
